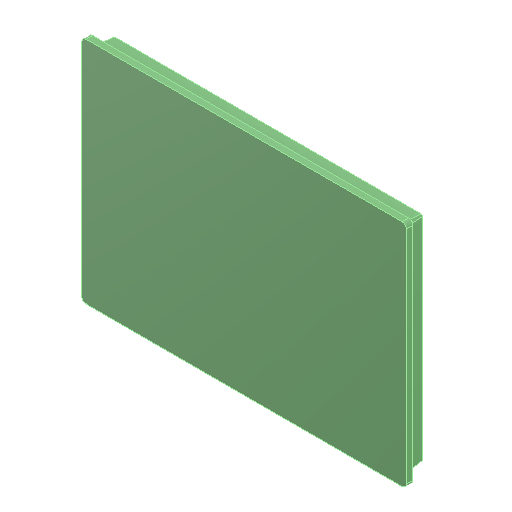
# Autodesk Inventor part: ImageToStl.com_82d01a97-71ed-4804-91bd-9032aadffd37
Saved by Autodesk Inventor 2026.1 (Build 301233020, 233B)
## iProperties
Created: 2026-02-19
Part Number: ImageToStl.com_82d01a97-71ed-4804-91bd-9032aadffd37
Material: Generic
Document SubType Name: Modeling
Designer: samuel
Density: 1 g/cm^3
Appearance: Smooth - Dark Forest Green
Author: samuel
Autodesk Inventor part; units mm, degrees
ref_plane "YZ Plane" through (0, 0, 0) normal (1, 0, 0) x (0, 1, 0)
ref_plane "XZ Plane" through (0, 0, 0) normal (0, 1, 0) x (-1, 0, 0)
ref_plane "XY Plane" through (0, 0, 0) normal (0, 0, 1) x (1, 0, 0)
sketch "Sketch1" plane through (0, 0, 0) normal (0, 0, 1) x (1, 0, 0)
  line L0 (-75, -53) -> (75, -53)
  line L1 (75, -53) -> (75, 53)
  line L2 (75, 53) -> (-75, 53)
  line L3 (-75, 53) -> (-75, -53)
  line L4 (-75, -53) -> (75, 53) construction
  line L5 (75, -53) -> (-75, 53) construction
  line L6 (-72, 50) -> (72, 50)
  line L7 (72, 50) -> (72, -50)
  line L8 (72, -50) -> (-72, -50)
  line L9 (-72, -50) -> (-72, 50)
  line L10 (69, 47) -> (-69, 47)
  line L11 (-69, 47) -> (-69, -47)
  line L12 (-69, -47) -> (69, -47)
  line L13 (69, -47) -> (69, 47)
  point P0 (0, 0)
  dimension "d0" = 150
  dimension "d1" = 106
  dimension "d4" = 3
  dimension "d5" = 3
  constraints: 28 end point, 6 parallel, 3 perpendicular, 2 midpoint, 1 horizontal, 6 other
  measures "d0" distance of L2.end L1.end
  measures "d1" distance of L1.end L0.end
  measures "d4" distance between parallel lines of L2 L6
  measures "d5" distance between parallel lines of L6 L10
extrude "Extrusion1" add sketch "Sketch1" along normal blind 3 contours L3 L2 L1 L0 | L6 L7 L8 L9 | L13 L12 L11 L10
extrude "Extrusion2" add sketch "Sketch1" against normal blind 8 contours L6 L7 L8 L9
fillet "Fillet1" radius 2 8 edges at (-75, 53, 1.5) (-69, 47, -4) (-75, -53, 1.5) (-69, -47, -4) (69, -47, -4) (75, -53, 1.5) (69, 47, -4) (75, 53, 1.5)
chamfer "Chamfer1" distance 1 angle 45 4 edges at (-72, -50, -4) (72, -50, -4) (72, 50, -4) (-72, 50, -4)
chamfer "Chamfer2" distance 0.5 distance2 5 8 edges at (72, 0, -8) (0, -50, -8) (-72, 0, -8) (0, 50, -8) (71.5, -49.5, -8) (-71.5, -49.5, -8) (-71.5, 49.5, -8) (71.5, 49.5, -8) measured on face at (22.3333, 49, -8)
body "Solid1"
